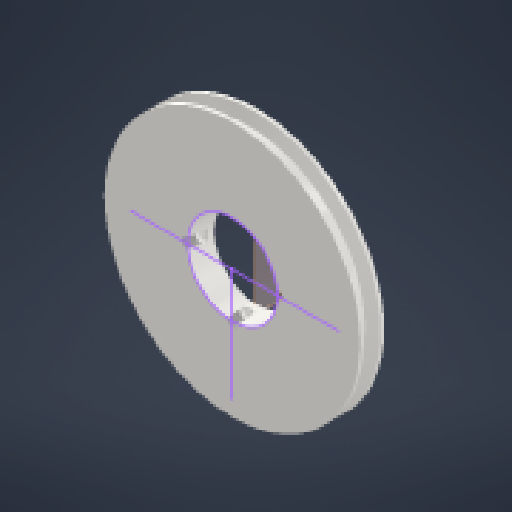
# Autodesk Inventor part: Poulie à gorge1
Saved by Autodesk Inventor 2026.2 (Build 302298010, 298A)
## iProperties
CustomPartVersion: 1
Created: 2026-03-31
Part Number: Poulie à gorge1
Material: Steel
Document SubType Name: Modeling
Designer: romai
Density: 1 g/cm^3
Appearance: Steel
Author: romai
Autodesk Inventor part; units mm, degrees
ref_plane "XZ Plane" through (0, 0, 0) normal (0, 1, 0) x (-1, 0, 0)
ref_plane "XY Plane" through (0, 0, 0) normal (0, 0, 1) x (1, 0, 0)
sketch "Esquisse principale" plane through (0, 0, 0) normal (1, 0, 0) x (0, 1, 0)
  line L0 (0, 22) -> (116.5, 22)
  line L1 (116.5, 22) -> (116.5, 18.6115)
  line L2 (116.5, 18.6115) -> (105.5, 15.2484)
  line L3 (105.5, 15.2484) -> (105.5, 6.7516)
  line L4 (105.5, 6.7516) -> (116.5, 3.3885)
  line L5 (116.5, 3.3885) -> (116.5, 0)
  line L6 (116.5, 0) -> (0, 0)
  line L7 (114.5, 18) -> (114.5, 4) construction
  line L8 (105.5, 11) -> (114.5, 11) construction
  line L9 (116.5, 18.6115) -> (116.5, 3.3885)
  line L10 (0, -4.4) -> (0, 26.4) projected
  line L11 (0, 0) -> (0, 22)
  dimension "d0" = 14
  dimension "d1" = 34
  dimension "d2" = 2
  dimension "d6" = 22
  dimension "d21" = 229
  dimension "d25" = 11
  dimension "d27" = 11
  constraints: 22 end point, 5 perpendicular, 2 collinear, 2 midpoint, 2 point on line, 1 parallel
  measures "d0" distance of L7.start L7.end
  measures "d1" angle of L2 L4
  measures "d2" distance between parallel lines of L1 L7
  measures "d6" distance between parallel lines of L6 L0
  measures "d21" diameter of L7 L10
  measures "d25" distance between parallel lines of L3 L9
  measures "d27" distance between parallel lines of L6 L8
ref_plane "Plan de courroie" through (0, 105.5, 11) normal (0, 0, 1) x (1, 0, 0)
revolve "Corps" add sketch "Esquisse principale" angle 360 about axis through (0, 0, -10) along (0, 0, 1)
revolve "Bord" cut sketch "Esquisse principale" angle 360 about axis through (0, 0, -10) along (0, 0, 1) contours L9 L4 L3 L2
fillet "Congé externe" [suppressed]
fillet "Congé interne" [suppressed]
sketch "Esquisse4" plane through (0, 0, 0) normal (1, 0, 0) x (0, 1, 0)
  line L0 (0, -20.2967) -> (0, 37.5815)
  line L1 (12.5, 32.25) -> (12.5, -12.25)
  line L2 (12.5, -12.25) -> (36.75, -12.25)
  line L3 (12.5, 32.25) -> (42.75, 32.25)
  line L4 (42.75, 32.25) -> (36.75, -12.25)
  line L5 (-116.5, 0) -> (116.5, 0) projected
  line L6 (12.5, 32.25) -> (0, 32.25)
  line L7 (12.5, -12.25) -> (0, -12.25)
  line L8 (0, -12.25) -> (0, 32.25)
  point P0 (0, 0)
  point P1 (0, 0)
  point P2 (12.5, 0)
  dimension "d48" = 12.5
  dimension "d49" = 73.5
  dimension "d50" = 85.5
  dimension "d51" = 44.5
  dimension "d52" = 12.25
  constraints: 16 end point, 2 horizontal, 2 perpendicular, 2 point on line, 2 vertical, 1 collinear, 1 parallel
  measures "d48" distance between parallel lines of L0 L1
  measures "d49" diameter of L2.end L0
  measures "d50" diameter of L3.end L0
  measures "d51" distance of L1.start L1.end
  measures "d52" distance between parallel lines of L5 L2
revolve "Révolution3" cut sketch "Esquisse4" angle 360 about axis through (0, 0, -20.2967) along (0, 0, 1) contours L0 L6 L1 L5 | L1 L5 L4 L2 | L1 L3 L4 L5
sketch "Esquisse5" plane through (0, 0, 22) normal (0, 0, 1) x (1, 0, 0)
  line L0 (0, 0) -> (97.3173, 0)
  line L1 (0, 0) -> (-92.8604, 0)
  line L2 (0, 0) -> (0, -102.459)
  circle A0 centre (0, 0) radius 40.9
  point P0 (0, 0)
  point P1 (0, -40.9)
  point P2 (-40.9051, 0)
  point P3 (40.9, 0)
  dimension "d68" = 81.8
  constraints: 6 end point, 3 point on line, 2 horizontal, 2 point on circle, 1 centre point, 1 coincident, 1 vertical
  measures "d68" diameter of A0
hole "Perçage3" at (0, -40.9, 22) at (-40.9051, 0, 22) at (40.9, 0, 22) direction (0, 0, -1) diameter 10.106 depth 15 tip angle 118 thread size "M12x1.75" class "6H" standard "ANSI Metric M Profile"
equation "\"d0\" = da_Bw"
equation "\"d1\" = da_Alfa"
equation "\"d2\" = da_c"
equation "\"d21\" = da_Dw"
equation "\"d25\" = da_Hd"
equation "\"d27\" = da_Se"
equation "\"da_r1\" = 0"
equation "\"da_r2\" = 0"
equation "\"d5\" = da_Se"
equation "\"da_Bw\" = 14"
equation "\"da_Alfa\" = 34deg"
equation "\"da_c\" = 2"
equation "\"da_Dw\" = 229"
equation "\"da_Hd\" = 11"
equation "\"da_Se\" = 11"
equation "\"da_Sg\" = 12"
body "Solid1"
